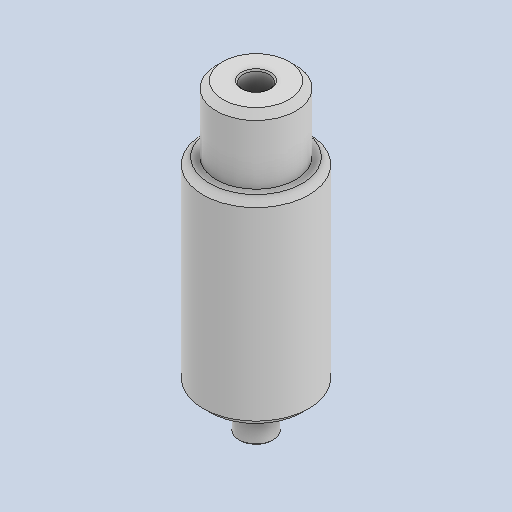
# Autodesk Inventor part: EPR Capillary Glue Ferrule
Saved by Autodesk Inventor 2025 (Build 290162010, 162A)
## iProperties
Created: 2024-11-14
Part Number: EPR Capillary Glue Ferrule
Material: Generic
Document SubType Name: Modeling
Designer: baas020
Density: 1 g/cm^3
Appearance: Default
Author: baas020
Autodesk Inventor part; units mm, degrees
ref_plane "YZ Plane" through (0, 0, 0) normal (1, 0, 0) x (0, 1, 0)
ref_plane "XZ Plane" through (0, 0, 0) normal (0, 1, 0) x (-1, 0, 0)
ref_plane "XY Plane" through (0, 0, 0) normal (0, 0, 1) x (1, 0, 0)
sketch "Sketch1" plane through (0, 0, 0) normal (0, 0, 1) x (1, 0, 0)
  line L0 (-3, 20) -> (-3, 15)
  line L1 (-3, 15) -> (-4, 15)
  line L2 (-4, 15) -> (-4, 0)
  line L3 (-1.3, 2) -> (-1.3, -3)
  line L4 (-1.3, -3) -> (-1, -3)
  line L5 (-1, -3) -> (-1, 20)
  line L6 (-1, 20) -> (-3, 20)
  line L7 (-1.3, 2) -> (-2.1, 2)
  line L8 (-2.1, 2) -> (-2.1, 0)
  line L9 (-2.1, 0) -> (-4, 0)
  line L10 (0, -7.6) -> (0, 24.6) projected
  point P0 (0, 0)
  dimension "d0" = 1
  dimension "d1" = 1.3
  dimension "d3" = 15
  dimension "d4" = 2
  dimension "d5" = 5
  dimension "d6" = 4
  dimension "d7" = 0.8
  dimension "d8" = 2
  dimension "d9" = 5
  constraints: 20 end point, 6 perpendicular, 3 vertical, 1 horizontal, 1 horizontal alignment
  measures "d0" distance from line of point (0, 0) L5
  measures "d1" distance from line of point (0, 0) L3
  measures "d3" distance of L1.end L2.end
  measures "d4" distance of L5.end L0.start
  measures "d5" distance of L0.start L0.end
  measures "d6" distance from line of point (0, 0) L2
  measures "d7" distance of L3.start L7.end
  measures "d8" distance of L7.end L8.end
  measures "d9" distance of L3.start L3.end
revolve "Revolution1" add sketch "Sketch1" angle 360 about axis through (0, -10, 0) along (0, 1, 0)
chamfer "Chamfer1" distance 0.5 angle 45 3 edges at (4, 15, 0) (3, 20, 0) (4, 0, 0)
chamfer "Chamfer2" distance 0.1 angle 45 4 edges at (2.1, 0, 0) (1.3, -3, 0) (1, -3, 0) (1, 20, 0)
body "Solid1"
